Autodesk Fusion 360 part; units mm, degrees
note: some values were not read from the file. Set by a fixed rule: which sketch regions a step uses.
(part 3 of 4)
sketch "Sketch1" plane through (0, 0, 0) normal (0, 1, 0) x (1, 0, 0) in component "Laser"
  line L0 (18.5, 76) -> (18.5, 71)
  line L1 (18.5, 71) -> (33.5, 71)
  line L2 (33.5, 71) -> (33.5, 76)
  line L3 (33.5, 76) -> (18.5, 76)
  circle A0 centre (44, 73.5) radius 3.5355
  circle A1 centre (14, 13) radius 3.5355
  line L4 (3, 87.5) -> (3, 72.5)
  line L5 (3, 72.5) -> (8, 72.5)
  line L6 (8, 72.5) -> (8, 87.5)
  line L7 (8, 87.5) -> (3, 87.5)
  line L8 (3, 37.5) -> (3, 19.5)
  line L9 (3, 19.5) -> (8, 19.5)
  line L10 (8, 19.5) -> (8, 37.5)
  line L11 (8, 37.5) -> (3, 37.5)
  line L12 (46.0207, 66) -> (42.2092, 66)
  arc A2 (42.2092, 66) -> (38.5894, 63.702) centre (42.2092, 62) ccw
  line L13 (38.5894, 63.702) -> (18.9309, 21.8917)
  arc A3 (18.9309, 21.8917) -> (19.0866, 18.1897) centre (22.5507, 20.1897) ccw
  line L14 (19.0866, 18.1897) -> (20.9282, 15)
  arc A4 (20.9282, 11) -> (20.9282, 15) centre (17.4641, 13) ccw
  line L15 (20.9282, 11) -> (19.1962, 8)
  arc A5 (15.7321, 6) -> (19.1962, 8) centre (15.7321, 10) ccw
  line L16 (15.7321, 6) -> (3, 6)
  arc A6 (0, 9) -> (3, 6) centre (3, 9) ccw
  line L17 (0, 9) -> (0, 42)
  arc A7 (1, 43) -> (0, 42) centre (1, 42) ccw
  arc A8 (1, 43) -> (3, 45) centre (1, 45) ccw
  line L18 (3, 45) -> (3, 66)
  arc A9 (3, 66) -> (1, 68) centre (1, 66) ccw
  arc A10 (0, 69) -> (1, 68) centre (1, 69) ccw
  line L19 (0, 69) -> (0, 103)
  arc A11 (3, 106) -> (0, 103) centre (3, 103) ccw
  line L20 (8, 106) -> (3, 106)
  line L21 (8, 106) -> (11.4183, 106)
  arc A12 (14.1539, 104.9183) -> (11.4183, 106) centre (11.4183, 102) ccw
  line L22 (14.1539, 104.9183) -> (38.5159, 82.0817)
  arc A13 (38.5159, 82.0817) -> (41.2515, 81) centre (41.2515, 85) ccw
  line L23 (41.2515, 81) -> (46.0207, 81)
  arc A14 (49.4848, 79) -> (46.0207, 81) centre (46.0207, 77) ccw
  line L24 (49.4848, 79) -> (51.5056, 75.5)
  arc A15 (51.5056, 71.5) -> (51.5056, 75.5) centre (48.0415, 73.5) ccw
  line L25 (51.5056, 71.5) -> (49.4848, 68)
  arc A16 (46.0207, 66) -> (49.4848, 68) centre (46.0207, 70) ccw
  line L26 (40.0053, -0.251) -> (40.0053, -5.251)
  line L27 (40.0053, -5.251) -> (25.0053, -5.251)
  line L28 (25.0053, -5.251) -> (25.0053, -0.251)
  line L29 (25.0053, -0.251) -> (40.0053, -0.251)
  circle A17 centre (14.5053, -2.751) radius 3.5355
  circle A18 centre (44.5053, 57.749) radius 3.5355
  line L30 (55.5053, -1.751) -> (55.5053, -16.751)
  line L31 (55.5053, -16.751) -> (50.5053, -16.751)
  line L32 (50.5053, -16.751) -> (50.5053, -1.751)
  line L33 (50.5053, -1.751) -> (55.5053, -1.751)
  line L34 (55.5053, 51.249) -> (55.5053, 33.249)
  line L35 (55.5053, 33.249) -> (50.5053, 33.249)
  line L36 (50.5053, 33.249) -> (50.5053, 51.249)
  line L37 (50.5053, 51.249) -> (55.5053, 51.249)
  line L38 (16.296, 4.749) -> (12.4845, 4.749)
  arc A19 (12.4845, 4.749) -> (9.0204, 2.749) centre (12.4845, 0.749) ccw
  line L39 (9.0204, 2.749) -> (6.9997, -0.751)
  arc A20 (6.9997, -0.751) -> (6.9997, -4.751) centre (10.4638, -2.751) ccw
  line L40 (6.9997, -4.751) -> (9.0204, -8.251)
  arc A21 (9.0204, -8.251) -> (12.4845, -10.251) centre (12.4845, -6.251) ccw
  line L41 (12.4845, -10.251) -> (17.2537, -10.251)
  arc A22 (19.9893, -11.3327) -> (17.2537, -10.251) centre (17.2537, -14.251) ccw
  line L42 (19.9893, -11.3327) -> (44.3513, -34.1693)
  arc A23 (44.3513, -34.1693) -> (47.0869, -35.251) centre (47.0869, -31.251) ccw
  line L43 (47.0869, -35.251) -> (50.5053, -35.251)
  line L44 (50.5053, -35.251) -> (55.5053, -35.251)
  arc A24 (55.5053, -35.251) -> (58.5053, -32.251) centre (55.5053, -32.251) ccw
  line L45 (58.5053, -32.251) -> (58.5053, 1.749)
  arc A25 (58.5053, 1.749) -> (57.5053, 2.749) centre (57.5053, 1.749) ccw
  arc A26 (55.5053, 4.749) -> (57.5053, 2.749) centre (57.5053, 4.749) ccw
  line L46 (55.5053, 4.749) -> (55.5053, 25.749)
  arc A27 (57.5053, 27.749) -> (55.5053, 25.749) centre (57.5053, 25.749) ccw
  arc A28 (57.5053, 27.749) -> (58.5053, 28.749) centre (57.5053, 28.749) ccw
  line L47 (58.5053, 28.749) -> (58.5053, 61.749)
  arc A29 (58.5053, 61.749) -> (55.5053, 64.749) centre (55.5053, 61.749) ccw
  line L48 (55.5053, 64.749) -> (42.7732, 64.749)
  arc A30 (42.7732, 64.749) -> (39.3091, 62.749) centre (42.7732, 60.749) ccw
  line L49 (39.3091, 62.749) -> (37.5771, 59.749)
  arc A31 (37.5771, 59.749) -> (37.5771, 55.749) centre (41.0412, 57.749) ccw
  line L50 (37.5771, 55.749) -> (39.4186, 52.5593)
  arc A32 (39.5744, 48.8573) -> (39.4186, 52.5593) centre (35.9545, 50.5593) ccw
  line L51 (39.5744, 48.8573) -> (19.9159, 7.047)
  arc A33 (16.296, 4.749) -> (19.9159, 7.047) centre (16.296, 8.749) ccw
  line L52 (-16.3164, 46.5423) -> (-30.7017, 46.5423)
  arc A34 (-16.3164, 46.5423) -> (-13.3678, 50.0951) centre (-16.3164, 49.5423) ccw
  line L53 (-15.2428, 60.0951) -> (-13.3678, 50.0951)
  arc A35 (-15.2428, 60.0951) -> (-18.1914, 62.5423) centre (-18.1914, 59.5423) ccw
  line L54 (-30.7017, 62.5423) -> (-18.1914, 62.5423)
  line L55 (-43.2119, 62.5423) -> (-30.7017, 62.5423)
  arc A36 (-43.2119, 62.5423) -> (-46.1605, 60.0951) centre (-43.2119, 59.5423) ccw
  line L56 (-48.0355, 50.0951) -> (-46.1605, 60.0951)
  arc A37 (-48.0355, 50.0951) -> (-45.0869, 46.5423) centre (-45.0869, 49.5423) ccw
  line L57 (-30.7017, 46.5423) -> (-45.0869, 46.5423)
  line L58 (-42.2017, 41.5423) -> (-42.2017, 36.5423)
  line L59 (-42.2017, 36.5423) -> (-19.2017, 36.5423)
  line L60 (-19.2017, 36.5423) -> (-19.2017, 41.5423)
  line L61 (-19.2017, 41.5423) -> (-42.2017, 41.5423)
  line L62 (-55.7017, 94.5423) -> (-55.7017, 106.5423)
  line L63 (-55.7017, 106.5423) -> (-47.7017, 106.5423)
  line L64 (-45.7017, 104.5423) -> (-45.7017, 97.6156)
  line L65 (-44.8073, 95.949) -> (-31.8073, 87.3248)
  line L66 (-29.596, 87.3248) -> (-16.596, 95.949)
  line L67 (-15.7017, 97.6156) -> (-15.7017, 104.5423)
  line L68 (-13.7017, 106.5423) -> (-5.7178, 106.5423)
  line L69 (-5.7178, 106.5423) -> (-5.7017, 94.5423)
  line L70 (-5.7017, 94.5423) -> (-5.7017, 93.0423)
  line L71 (-5.7017, 93.0423) -> (-0.7017, 93.0423)
  line L72 (-0.7017, 93.0423) -> (-0.7017, 75.0423)
  line L73 (-0.7017, 75.0423) -> (-5.7017, 75.0423)
  line L74 (-5.7017, 75.0423) -> (-5.7017, 40.0423)
  line L75 (-5.7017, 40.0423) -> (-0.7017, 40.0423)
  line L76 (-0.7017, 40.0423) -> (-0.7017, 25.0423)
  line L77 (-0.7017, 25.0423) -> (-5.7017, 25.0423)
  line L78 (-5.7017, 25.0423) -> (-5.7017, 6.5423)
  line L79 (-5.7017, 6.5423) -> (-55.7017, 6.5423)
  line L80 (-55.7017, 6.5423) -> (-55.7017, 25.0423)
  line L81 (-55.7017, 25.0423) -> (-60.7017, 25.0423)
  line L82 (-60.7017, 25.0423) -> (-60.7017, 40.0423)
  line L83 (-60.7017, 40.0423) -> (-55.7017, 40.0423)
  line L84 (-55.7017, 40.0423) -> (-55.7017, 75.0423)
  line L85 (-55.7017, 75.0423) -> (-60.7017, 75.0423)
  line L86 (-60.7017, 75.0423) -> (-60.7017, 93.0423)
  line L87 (-60.7017, 93.0423) -> (-55.7017, 93.0423)
  line L88 (-55.7017, 93.0423) -> (-55.7017, 94.5423)
  line L89 (-2.7161, 5.444) -> (-0.1384, 4.2894)
  line L90 (-0.1384, 4.2894) -> (4.8616, 4.2894)
  spline S0 degree 2 poles (5.8616, 3.3935) (5.8616, 4.2894) (4.8616, 4.2894) knots -112.214913 -112.214913 -112.214913 -110.644117 -110.644117 -110.644117 weights 1 0.707107 1
  line L91 (5.8616, 3.3935) -> (5.8616, 0.7057)
  spline S1 degree 2 poles (4.8616, -0.1902) (5.8616, -0.1902) (5.8616, 0.7057) knots -116.78571 -116.78571 -116.78571 -115.214913 -115.214913 -115.214913 weights 1 0.707107 1
  line L92 (4.8616, -0.1902) -> (-0.1384, -0.1902)
  line L93 (-0.1384, -0.1902) -> (-2.7161, -1.3448)
  spline S2 degree 2 poles (-3.6105, -1.534) (-3.1384, -1.534) (-2.7161, -1.3448) knots -125.594971 -125.594971 -125.594971 -124.667676 -124.667676 -124.667676 weights 1 0.973249 1
  line L94 (-3.6105, -1.534) -> (-11.1384, -1.534)
  spline S3 degree 2 poles (-13.1384, -3.3258) (-13.1384, -1.534) (-11.1384, -1.534) knots -136.264428 -136.264428 -136.264428 -133.122835 -133.122835 -133.122835 weights 1 0.707107 1
  line L95 (-13.1384, -3.3258) -> (-13.1384, -8.7012)
  spline S4 degree 2 poles (-15.1384, -10.493) (-13.1384, -10.493) (-13.1384, -8.7012) knots -145.40602 -145.40602 -145.40602 -142.264428 -142.264428 -142.264428 weights 1 0.707107 1
  line L96 (-15.1384, -10.493) -> (-35.1384, -10.493)
  spline S5 degree 2 poles (-37.1384, -8.7012) (-37.1384, -10.493) (-35.1384, -10.493) knots -9.783185 -9.783185 -9.783185 -6.641593 -6.641593 -6.641593 weights 1 0.707107 1
  line L97 (-37.1384, -8.7012) -> (-37.1384, -3.3258)
  spline S6 degree 2 poles (-39.1384, -1.534) (-37.1384, -1.534) (-37.1384, -3.3258) knots -18.924778 -18.924778 -18.924778 -15.783185 -15.783185 -15.783185 weights 1 0.707107 1
  line L98 (-39.1384, -1.534) -> (-46.6663, -1.534)
  spline S7 degree 2 poles (-47.5607, -1.3448) (-47.1384, -1.534) (-46.6663, -1.534) knots -27.379937 -27.379937 -27.379937 -26.452642 -26.452642 -26.452642 weights 1 0.973249 1
  line L99 (-47.5607, -1.3448) -> (-50.1384, -0.1902)
  line L100 (-50.1384, -0.1902) -> (-55.1384, -0.1902)
  spline S8 degree 2 poles (-56.1384, 0.7057) (-56.1384, -0.1902) (-55.1384, -0.1902) knots -36.8327 -36.8327 -36.8327 -35.261903 -35.261903 -35.261903 weights 1 0.707107 1
  line L101 (-56.1384, 0.7057) -> (-56.1384, 3.3935)
  spline S9 degree 2 poles (-55.1384, 4.2894) (-56.1384, 4.2894) (-56.1384, 3.3935) knots -41.403496 -41.403496 -41.403496 -39.8327 -39.8327 -39.8327 weights 1 0.707107 1
  line L102 (-55.1384, 4.2894) -> (-50.1384, 4.2894)
  line L103 (-50.1384, 4.2894) -> (-47.5607, 5.444)
  spline S10 degree 2 poles (-46.6663, 5.6332) (-47.1384, 5.6332) (-47.5607, 5.444) knots -50.212757 -50.212757 -50.212757 -49.285462 -49.285462 -49.285462 weights 1 0.973249 1
  line L104 (-46.6663, 5.6332) -> (-34.1384, 5.6332)
  spline S11 degree 2 poles (-32.1384, 3.8414) (-32.1384, 5.6332) (-34.1384, 5.6332) knots -65.882214 -65.882214 -65.882214 -62.740621 -62.740621 -62.740621 weights 1 0.707107 1
  line L105 (-32.1384, 3.8414) -> (-32.1384, 0.2578)
  line L106 (-32.1384, 0.2578) -> (-18.1384, 0.2578)
  line L107 (-18.1384, 0.2578) -> (-18.1384, 3.8414)
  spline S12 degree 2 poles (-16.1384, 5.6332) (-18.1384, 5.6332) (-18.1384, 3.8414) knots -89.306992 -89.306992 -89.306992 -86.165399 -86.165399 -86.165399 weights 1 0.707107 1
  line L108 (-16.1384, 5.6332) -> (-3.6105, 5.6332)
  spline S13 degree 2 poles (-2.7161, 5.444) (-3.1384, 5.6332) (-3.6105, 5.6332) knots -102.762151 -102.762151 -102.762151 -101.834856 -101.834856 -101.834856 weights 1 0.973249 1
  arc A38 (-40.8714, -17.6968) -> (-38.5209, -18.8326) centre (-38.5209, -15.8326) ccw
  line L109 (-38.5209, -18.8326) -> (-14.4202, -18.8326)
  arc A39 (-14.4202, -18.8326) -> (-12.0697, -17.6968) centre (-14.4202, -15.8326) ccw
  line L110 (-1.4705, -4.3326) -> (3.5295, -4.3326)
  line L111 (3.5295, -4.3326) -> (3.5295, -19.3326)
  line L112 (3.5295, -19.3326) -> (-1.4705, -19.3326)
  line L113 (-1.4705, -19.3326) -> (-1.4705, -29.8326)
  line L114 (-1.4705, -29.8326) -> (-14.9705, -29.8326)
  line L115 (-14.9705, -29.8326) -> (-14.9705, -34.8326)
  line L116 (-14.9705, -34.8326) -> (-37.9705, -34.8326)
  line L117 (-37.9705, -34.8326) -> (-37.9705, -29.8326)
  line L118 (-37.9705, -29.8326) -> (-51.4705, -29.8326)
  line L119 (-51.4705, -29.8326) -> (-51.4705, -19.3326)
  line L120 (-51.4705, -19.3326) -> (-56.4705, -19.3326)
  line L121 (-56.4705, -19.3326) -> (-56.4705, -4.3326)
  line L122 (-56.4705, -4.3326) -> (-51.4705, -4.3326)
  line L123 (-51.4705, -4.3326) -> (-51.4705, -2.497)
  line L124 (-51.4705, -2.497) -> (-49.8826, -2.497)
  line L125 (-49.8826, -2.497) -> (-40.8714, -17.6968)
  line L126 (-12.0697, -17.6968) -> (-2.8826, -2.497)
  line L127 (-2.8826, -2.497) -> (-1.4705, -2.497)
  line L128 (-1.4705, -2.497) -> (-1.4705, -4.3326)
  line L129 (24.5846, -33.7494) -> (32.307, -41.9317)
  arc A40 (24.5846, -33.7494) -> (21.1301, -35.1221) centre (23.1301, -35.1221) ccw
  line L130 (21.1301, -43.3044) -> (21.1301, -35.1221)
  arc A41 (21.1301, -43.3044) -> (23.1301, -45.3044) centre (23.1301, -43.3044) ccw
  line L131 (30.8524, -45.3044) -> (23.1301, -45.3044)
  arc A42 (30.8524, -45.3044) -> (32.307, -41.9317) centre (30.8524, -43.3044) ccw
  arc A43 (-11.9711, -41.4934) -> (-11.1225, -45.3044) centre (-11.1225, -43.3044) ccw
  line L132 (-2.6294, -45.3044) -> (-11.1225, -45.3044)
  arc A44 (-2.6294, -45.3044) -> (-1.9491, -41.4237) centre (-2.6294, -43.3044) ccw
  line L133 (-6.7423, -39.69) -> (-1.9491, -41.4237)
  arc A45 (-6.7423, -39.69) -> (-8.2711, -39.7597) centre (-7.4225, -41.5707) ccw
  line L134 (-11.9711, -41.4934) -> (-8.2711, -39.7597)
  line L135 (13.4498, -41.6765) -> (3.4244, -38.0502)
  arc A46 (13.4498, -41.6765) -> (16.1301, -39.7957) centre (14.1301, -39.7957) ccw
  line L136 (16.1301, -31.4719) -> (16.1301, -39.7957)
  arc A47 (16.1301, -31.4719) -> (13.2815, -29.6609) centre (14.1301, -31.4719) ccw
  line L137 (3.256, -34.3584) -> (13.2815, -29.6609)
  arc A48 (3.256, -34.3584) -> (3.4244, -38.0502) centre (4.1046, -36.1695) ccw
  line L138 (-8.2711, -55.8492) -> (-11.9711, -54.1155)
  arc A49 (-8.2711, -55.8492) -> (-6.7423, -55.9189) centre (-7.4225, -54.0381) ccw
  line L139 (-1.9491, -54.1852) -> (-6.7423, -55.9189)
  arc A50 (-1.9491, -54.1852) -> (-2.6294, -50.3044) centre (-2.6294, -52.3044) ccw
  line L140 (-11.1225, -50.3044) -> (-2.6294, -50.3044)
  arc A51 (-11.1225, -50.3044) -> (-11.9711, -54.1155) centre (-11.1225, -52.3044) ccw
  arc A52 (13.2815, -65.948) -> (16.1301, -64.137) centre (14.1301, -64.137) ccw
  line L141 (16.1301, -55.8131) -> (16.1301, -64.137)
  arc A53 (16.1301, -55.8131) -> (13.4498, -53.9324) centre (14.1301, -55.8131) ccw
  line L142 (3.4244, -57.5586) -> (13.4498, -53.9324)
  arc A54 (3.4244, -57.5586) -> (3.256, -61.2504) centre (4.1046, -59.4394) ccw
  line L143 (13.2815, -65.948) -> (3.256, -61.2504)
  line L144 (21.1301, -60.4867) -> (21.1301, -52.3044)
  arc A55 (21.1301, -60.4867) -> (24.5846, -61.8595) centre (23.1301, -60.4867) ccw
  line L145 (32.307, -53.6772) -> (24.5846, -61.8595)
  arc A56 (32.307, -53.6772) -> (30.8524, -50.3044) centre (30.8524, -52.3044) ccw
  line L146 (23.1301, -50.3044) -> (30.8524, -50.3044)
  arc A57 (23.1301, -50.3044) -> (21.1301, -52.3044) centre (23.1301, -52.3044) ccw
  circle A58 centre (-35.1347, -47.8044) radius 0.375
  spline S14 degree 2 poles (20.1301, -78.8044) (21.1301, -78.8044) (21.1301, -77.8044) (21.1301, -75.3044) (21.1301, -72.8044) knots -186.864147 -186.864147 -186.864147 -185.29335 -185.29335 -180.29335 -180.29335 -180.29335 weights 1 0.707107 1 1 1
  line L147 (20.1301, -78.8044) -> (17.177, -78.8044)
  line L148 (17.1301, -78.8044) -> (17.177, -78.8044)
  spline S15 degree 2 poles (17.1301, -16.8044) (16.1301, -16.8044) (16.1301, -17.8044) (16.1301, -20.3044) (16.1301, -22.8044) knots -57.72942 -57.72942 -57.72942 -56.158624 -56.158624 -51.158624 -51.158624 -51.158624 weights 1 0.707107 1 1 1
  line L149 (20.1301, -16.8044) -> (17.1301, -16.8044)
  spline S16 degree 2 poles (21.1301, -22.8044) (21.1301, -20.3044) (21.1301, -17.8044) (21.1301, -16.8044) (20.1301, -16.8044) knots -67.300216 -67.300216 -67.300216 -62.300216 -62.300216 -60.72942 -60.72942 -60.72942 weights 1 1 1 0.707107 1
  spline S17 degree 2 poles (21.1301, -72.8044) (30.0204, -63.3846) (38.9108, -53.9647) (39.8424, -52.9775) (41.1039, -53.4788) (42.3653, -53.9801) (42.3653, -55.3374) (42.3653, -56.5709) (42.3653, -57.8044) (42.3653, -58.8044) (43.3653, -58.8044) (44.8653, -58.8044) (46.3653, -58.8044) (47.3653, -58.8044) (47.3653, -57.8044) (47.3653, -55.0544) (47.3653, -52.3044) (47.3653, -50.3044) (49.3653, -50.3044) (52.1153, -50.3044) (54.8653, -50.3044) (55.8653, -50.3044) (55.8653, -49.3044) (55.8653, -47.8044) (55.8653, -46.3044) (55.8653, -45.3044) (54.8653, -45.3044) (52.1153, -45.3044) (49.3653, -45.3044) (47.3653, -45.3044) (47.3653, -43.3044) (47.3653, -40.5544) (47.3653, -37.8044) (47.3653, -36.8044) (46.3653, -36.8044) (44.8653, -36.8044) (43.3653, -36.8044) (42.3653, -36.8044) (42.3653, -37.8044) (42.3653, -39.0379) (42.3653, -40.2714) (42.3653, -41.6288) (41.1039, -42.1301) (39.8424, -42.6313) (38.9108, -41.6442) (30.0204, -32.2243) (21.1301, -22.8044) knots -180.29335 -180.29335 -180.29335 -154.387975 -154.387975 -152.002869 -152.002869 -149.617763 -149.617763 -147.150765 -147.150765 -145.579969 -145.579969 -142.579969 -142.579969 -141.009172 -141.009172 -135.509172 -135.509172 -132.36758 -132.36758 -126.86758 -126.86758 -125.296783 -125.296783 -122.296783 -122.296783 -120.725987 -120.725987 -115.225987 -115.225987 -112.084394 -112.084394 -106.584394 -106.584394 -105.013598 -105.013598 -102.013598 -102.013598 -100.442802 -100.442802 -97.975804 -97.975804 -95.590698 -95.590698 -93.205592 -93.205592 -67.300216 -67.300216 -67.300216 weights 1 1 1 0.827432 1 0.827432 1 1 1 0.707107 1 1 1 0.707107 1 1 1 0.707107 1 1 1 0.707107 1 1 1 0.707107 1 1 1 0.707107 1 1 1 0.707107 1 1 1 0.707107 1 1 1 0.827432 1 0.827432 1 1 1
  line L150 (-47.8995, -42.8044) -> (-45.3836, -42.8044)
  line L151 (-44.4198, -42.5569) -> (-35.8866, -37.8636)
  line L152 (-33.8798, -37.9095) -> (-26.7944, -42.2394)
  line L153 (-24.8917, -42.3386) -> (16.1301, -22.8044)
  spline S18 degree 2 poles (16.1301, -72.8044) (16.1301, -75.3044) (16.1301, -77.8044) (16.1301, -78.8044) (17.1301, -78.8044) knots -196.434943 -196.434943 -196.434943 -191.434943 -191.434943 -189.864147 -189.864147 -189.864147 weights 1 1 1 0.707107 1
  line L154 (-24.8917, -53.2703) -> (16.1301, -72.8044)
  line L155 (-33.8798, -57.6994) -> (-26.7944, -53.3694)
  line L156 (-44.4198, -53.052) -> (-35.8866, -57.7453)
  line L157 (-47.8995, -52.8044) -> (-45.3836, -52.8044)
  line L158 (-49.8995, -44.8044) -> (-49.8995, -50.8044)
  arc A59 (-44.4198, -53.052) -> (-45.3836, -52.8044) centre (-45.3836, -54.8044) ccw
  arc A60 (-45.3836, -42.8044) -> (-44.4198, -42.5569) centre (-45.3836, -40.8044) ccw
  arc A61 (-47.8995, -42.8044) -> (-49.8995, -44.8044) centre (-47.8995, -44.8044) ccw
  arc A62 (-33.8798, -37.9095) -> (-35.8866, -37.8636) centre (-34.9227, -39.616) ccw
  arc A63 (-26.7944, -42.2394) -> (-24.8917, -42.3386) centre (-25.7515, -40.5329) ccw
  arc A64 (-24.8917, -53.2703) -> (-26.7944, -53.3694) centre (-25.7515, -55.076) ccw
  arc A65 (-35.8866, -57.7453) -> (-33.8798, -57.6994) centre (-34.9227, -55.9928) ccw
  arc A66 (-49.8995, -50.8044) -> (-47.8995, -52.8044) centre (-47.8995, -50.8044) ccw
  line L159 (-48.7017, 18.4806) -> (-48.7017, 14.5423)
  line L160 (-46.7017, 12.5423) -> (-41.5819, 12.5423)
  line L161 (-40.3625, 16.1275) -> (-45.4822, 20.0658)
  line L162 (-47.7017, 83.6559) -> (-47.7017, 69.5423)
  line L163 (-45.7017, 67.5423) -> (-35.7017, 67.5423)
  line L164 (-33.7017, 69.5423) -> (-33.7017, 76.513)
  line L165 (-34.5392, 78.1405) -> (-44.5392, 85.2834)
  line L166 (-25.7017, 29.5423) -> (-25.7017, 21.6316)
  line L167 (-22.4738, 20.0529) -> (-12.3029, 27.9636)
  line L168 (-13.5307, 31.5423) -> (-23.7017, 31.5423)
  line L169 (-15.9211, 20.0658) -> (-21.0408, 16.1275)
  line L170 (-19.8214, 12.5423) -> (-14.7017, 12.5423)
  line L171 (-12.7017, 14.5423) -> (-12.7017, 18.4806)
  line L172 (-27.7017, 76.513) -> (-27.7017, 69.5423)
  line L173 (-25.7017, 67.5423) -> (-15.7017, 67.5423)
  line L174 (-13.7017, 69.5423) -> (-13.7017, 83.6559)
  line L175 (-16.8641, 85.2834) -> (-26.8641, 78.1405)
  line L176 (-49.1005, 27.9636) -> (-38.9295, 20.0529)
  line L177 (-35.7017, 21.6316) -> (-35.7017, 29.5423)
  line L178 (-37.7017, 31.5423) -> (-47.8726, 31.5423)
  arc A67 (-48.7017, 14.5423) -> (-46.7017, 12.5423) centre (-46.7017, 14.5423) ccw
  arc A68 (-41.5819, 12.5423) -> (-40.3625, 16.1275) centre (-41.5819, 14.5423) ccw
  arc A69 (-45.4822, 20.0658) -> (-48.7017, 18.4806) centre (-46.7017, 18.4806) ccw
  arc A70 (-47.7017, 69.5423) -> (-45.7017, 67.5423) centre (-45.7017, 69.5423) ccw
  arc A71 (-35.7017, 67.5423) -> (-33.7017, 69.5423) centre (-35.7017, 69.5423) ccw
  arc A72 (-33.7017, 76.513) -> (-34.5392, 78.1405) centre (-35.7017, 76.513) ccw
  arc A73 (-44.5392, 85.2834) -> (-47.7017, 83.6559) centre (-45.7017, 83.6559) ccw
  arc A74 (-25.7017, 21.6316) -> (-22.4738, 20.0529) centre (-23.7017, 21.6316) ccw
  arc A75 (-12.3029, 27.9636) -> (-13.5307, 31.5423) centre (-13.5307, 29.5423) ccw
  arc A76 (-23.7017, 31.5423) -> (-25.7017, 29.5423) centre (-23.7017, 29.5423) ccw
  arc A77 (-21.0408, 16.1275) -> (-19.8214, 12.5423) centre (-19.8214, 14.5423) ccw
  arc A78 (-14.7017, 12.5423) -> (-12.7017, 14.5423) centre (-14.7017, 14.5423) ccw
  arc A79 (-12.7017, 18.4806) -> (-15.9211, 20.0658) centre (-14.7017, 18.4806) ccw
  arc A80 (-27.7017, 69.5423) -> (-25.7017, 67.5423) centre (-25.7017, 69.5423) ccw
  arc A81 (-15.7017, 67.5423) -> (-13.7017, 69.5423) centre (-15.7017, 69.5423) ccw
  arc A82 (-13.7017, 83.6559) -> (-16.8641, 85.2834) centre (-15.7017, 83.6559) ccw
  arc A83 (-26.8641, 78.1405) -> (-27.7017, 76.513) centre (-25.7017, 76.513) ccw
  arc A84 (-38.9295, 20.0529) -> (-35.7017, 21.6316) centre (-37.7017, 21.6316) ccw
  arc A85 (-35.7017, 29.5423) -> (-37.7017, 31.5423) centre (-37.7017, 29.5423) ccw
  arc A86 (-47.8726, 31.5423) -> (-49.1005, 27.9636) centre (-47.8726, 29.5423) ccw
  arc A87 (-45.7017, 104.5423) -> (-47.7017, 106.5423) centre (-47.7017, 104.5423) ccw
  arc A88 (-45.7017, 97.6156) -> (-44.8073, 95.949) centre (-43.7017, 97.6156) ccw
  arc A89 (-31.8073, 87.3248) -> (-29.596, 87.3248) centre (-30.7017, 88.9914) ccw
  arc A90 (-16.596, 95.949) -> (-15.7017, 97.6156) centre (-17.7017, 97.6156) ccw
  arc A91 (-13.7017, 106.5423) -> (-15.7017, 104.5423) centre (-13.7017, 104.5423) ccw
  arc A92 (16.6636, 53.9448) -> (12, 52.6922) centre (14.5, 52.6922) ccw
  line L179 (12, 52.6922) -> (12, 31.0216)
  arc A93 (12, 31.0216) -> (16.7553, 29.943) centre (14.5, 31.0216) ccw
  line L180 (16.7553, 29.943) -> (22.431, 41.8102)
  arc A94 (22.431, 41.8102) -> (22.3392, 44.1414) centre (20.1756, 42.8888) ccw
  line L181 (22.3392, 44.1414) -> (16.6636, 53.9448)
  arc A95 (23.5394, 52.2182) -> (27.9834, 52.4625) centre (25.6988, 53.4779) ccw
  line L182 (27.9834, 52.4625) -> (32.4376, 62.4847)
  arc A96 (32.4376, 62.4847) -> (30.1531, 66) centre (30.1531, 63.5) ccw
  line L183 (30.1531, 66) -> (19.8526, 66)
  arc A97 (19.8526, 66) -> (17.6931, 62.2403) centre (19.8526, 63.5) ccw
  line L184 (17.6931, 62.2403) -> (23.5394, 52.2182)
  arc A98 (12, 83.5) -> (14.5, 81) centre (14.5, 83.5) ccw
  line L185 (14.5, 81) -> (26.1249, 81)
  arc A99 (26.1249, 81) -> (27.8243, 85.3336) centre (26.1249, 83.5) ccw
  line L186 (27.8243, 85.3336) -> (16.1994, 96.1079)
  arc A100 (16.1994, 96.1079) -> (12, 94.2743) centre (14.5, 94.2743) ccw
  line L187 (12, 94.2743) -> (12, 83.5)
  line L188 (41.8417, 16.8043) -> (36.1661, 26.6076)
  arc A101 (36.0743, 28.9389) -> (36.1661, 26.6076) centre (38.3296, 27.8602) ccw
  line L189 (36.0743, 28.9389) -> (41.7499, 40.8061)
  arc A102 (46.5053, 39.7274) -> (41.7499, 40.8061) centre (44.0053, 39.7274) ccw
  line L190 (46.5053, 39.7274) -> (46.5053, 18.0569)
  arc A103 (41.8417, 16.8043) -> (46.5053, 18.0569) centre (44.0053, 18.0569) ccw
  line L191 (34.9659, 18.5308) -> (40.8121, 8.5087)
  arc A104 (38.6527, 4.749) -> (40.8121, 8.5087) centre (38.6527, 7.249) ccw
  line L192 (38.6527, 4.749) -> (28.3522, 4.749)
  arc A105 (26.0676, 8.2644) -> (28.3522, 4.749) centre (28.3522, 7.249) ccw
  line L193 (26.0676, 8.2644) -> (30.5219, 18.2865)
  arc A106 (34.9659, 18.5308) -> (30.5219, 18.2865) centre (32.8064, 17.2711) ccw
  line L194 (46.5053, -12.751) -> (46.5053, -23.5253)
  arc A107 (42.3059, -25.3588) -> (46.5053, -23.5253) centre (44.0053, -23.5253) ccw
  line L195 (42.3059, -25.3588) -> (30.681, -14.5845)
  arc A108 (32.3804, -10.251) -> (30.681, -14.5845) centre (32.3804, -12.751) ccw
  line L196 (32.3804, -10.251) -> (44.0053, -10.251)
  arc A109 (46.5053, -12.751) -> (44.0053, -10.251) centre (44.0053, -12.751) ccw
  line L197 (-6.0029, 6.9715) -> (-55, 7) construction
  line L198 (-55, 7) -> (-54.9971, 12.0285) construction
  line L199 (-54.9971, 12.0285) -> (-6, 12) construction
  line L200 (-6, 12) -> (-6.0029, 6.9715) construction
  line L201 (-1.5502, -47.9713) -> (-1.5877, -47.8678)
  line L202 (-1.5877, -47.8678) -> (-1.4719, -47.8496)
  line L203 (-1.4719, -47.8496) -> (-1.5367, -47.7594)
  line L204 (-1.5367, -47.7594) -> (-1.4303, -47.7129)
  line L205 (-1.4303, -47.7129) -> (-1.5191, -47.642)
  line L206 (-1.5191, -47.642) -> (-1.4303, -47.5707)
  line L207 (-1.4303, -47.5707) -> (-1.5367, -47.5246)
  line L208 (-1.5367, -47.5246) -> (-1.4719, -47.4338)
  line L209 (-1.4719, -47.4338) -> (-1.5877, -47.4158)
  line L210 (-1.5877, -47.4158) -> (-1.5502, -47.3127)
  line L211 (-1.5502, -47.3127) -> (-1.6672, -47.324)
  line L212 (-1.6672, -47.324) -> (-1.6631, -47.2156)
  line L213 (-1.6631, -47.2156) -> (-1.7723, -47.2557)
  line L214 (-1.7723, -47.2557) -> (-1.8, -47.1504)
  line L215 (-1.8, -47.1504) -> (-1.8934, -47.216)
  line L216 (-1.8934, -47.216) -> (-1.9508, -47.1215)
  line L217 (-1.9508, -47.1215) -> (-2.0217, -47.208)
  line L218 (-2.0217, -47.208) -> (-2.1045, -47.1309)
  line L219 (-2.1045, -47.1309) -> (-2.1473, -47.232)
  line L220 (-2.1473, -47.232) -> (-2.2496, -47.1785)
  line L221 (-2.2496, -47.1785) -> (-2.2611, -47.2865)
  line L222 (-2.2611, -47.2865) -> (-2.3756, -47.2605)
  line L223 (-2.3756, -47.2605) -> (-2.3553, -47.3674)
  line L224 (-2.3553, -47.3674) -> (-2.473, -47.3709)
  line L225 (-2.473, -47.3709) -> (-2.4221, -47.4687)
  line L226 (-2.4221, -47.4687) -> (-2.5346, -47.501)
  line L227 (-2.5346, -47.501) -> (-2.457, -47.5826)
  line L228 (-2.457, -47.5826) -> (-2.5557, -47.642)
  line L229 (-2.5557, -47.642) -> (-2.457, -47.7012)
  line L230 (-2.457, -47.7012) -> (-2.5346, -47.7826)
  line L231 (-2.5346, -47.7826) -> (-2.4221, -47.8152)
  line L232 (-2.4221, -47.8152) -> (-2.473, -47.9131)
  line L233 (-2.473, -47.9131) -> (-2.3553, -47.9164)
  line L234 (-2.3553, -47.9164) -> (-2.3756, -48.0232)
  line L235 (-2.3756, -48.0232) -> (-2.2611, -47.9971)
  line L236 (-2.2611, -47.9971) -> (-2.2496, -48.1055)
  line L237 (-2.2496, -48.1055) -> (-2.1473, -48.0518)
  line L238 (-2.1473, -48.0518) -> (-2.1045, -48.1527)
  line L239 (-2.1045, -48.1527) -> (-2.0217, -48.0758)
  line L240 (-2.0217, -48.0758) -> (-1.9508, -48.1625)
  line L241 (-1.9508, -48.1625) -> (-1.8934, -48.0676)
  line L242 (-1.8934, -48.0676) -> (-1.8, -48.1336)
  line L243 (-1.8, -48.1336) -> (-1.7723, -48.0281)
  line L244 (-1.7723, -48.0281) -> (-1.6631, -48.0684)
  line L245 (-1.6631, -48.0684) -> (-1.6672, -47.9596)
  line L246 (-1.6672, -47.9596) -> (-1.5502, -47.9713)
  line L247 (-2.252, -46.9203) -> (-2.2019, -46.9133)
  line L248 (-2.2019, -46.9133) -> (-2.166, -46.907)
  line L249 (-2.166, -46.907) -> (-1.9846, -46.9019)
  line L250 (-1.9846, -46.9019) -> (-1.8055, -46.9328)
  line L251 (-1.8055, -46.9328) -> (-1.7707, -46.9441)
  line L252 (-1.7707, -46.9441) -> (-1.7485, -46.9508)
  line L253 (-1.7485, -46.9508) -> (-1.6305, -46.9992)
  line L254 (-1.6305, -46.9992) -> (-1.4746, -47.0762)
  line L255 (-1.4746, -47.0762) -> (-1.4332, -47.0971)
  line L256 (-1.4332, -47.0971) -> (-1.4111, -47.1084)
  line L257 (-1.4111, -47.1084) -> (-1.3451, -47.1436)
  line L258 (-1.3451, -47.1436) -> (-1.2879, -47.175)
  line L259 (-1.2879, -47.175) -> (-1.2416, -47.1982)
  line L260 (-1.2416, -47.1982) -> (-1.2008, -47.2148)
  line L261 (-1.2008, -47.2148) -> (-1.1869, -47.2197)
  line L262 (-1.1869, -47.2197) -> (-1.1623, -47.2287)
  line L263 (-1.1623, -47.2287) -> (-0.9057, -47.2801)
  line L264 (-0.9057, -47.2801) -> (-0.8793, -47.2812)
  line L265 (-0.8793, -47.2812) -> (-0.7868, -47.2812)
  line L266 (-0.7868, -47.2812) -> (-0.5756, -47.2853)
  line L267 (-0.5756, -47.2853) -> (-0.5756, -48.0803)
  line L268 (-0.5756, -48.0803) -> (-0.8482, -48.0781)
  line L269 (-0.8482, -48.0781) -> (-0.8822, -48.0795)
  line L270 (-0.8822, -48.0795) -> (-1.2161, -48.1305)
  line L271 (-1.2161, -48.1305) -> (-1.2486, -48.1393)
  line L272 (-1.2486, -48.1393) -> (-1.2494, -48.1396)
  line L273 (-1.2494, -48.1396) -> (-1.258, -48.143)
  line L274 (-1.258, -48.143) -> (-1.2611, -48.143)
  line L275 (-1.2611, -48.143) -> (-1.2818, -48.149)
  line L276 (-1.2818, -48.149) -> (-1.474, -48.243)
  line L277 (-1.474, -48.243) -> (-1.4914, -48.2555)
  line L278 (-1.4914, -48.2555) -> (-1.5191, -48.274)
  line L279 (-1.5191, -48.274) -> (-1.6662, -48.3498)
  line L280 (-1.6662, -48.3498) -> (-1.823, -48.4021)
  line L281 (-1.823, -48.4021) -> (-1.8555, -48.4088)
  line L282 (-1.8555, -48.4088) -> (-1.8803, -48.4135)
  line L283 (-1.8803, -48.4135) -> (-2.1307, -48.4135)
  line L284 (-2.1307, -48.4135) -> (-2.1555, -48.4088)
  line L285 (-2.1555, -48.4088) -> (-2.1758, -48.4049)
  line L286 (-2.1758, -48.4049) -> (-2.3686, -48.3334)
  line L287 (-2.3686, -48.3334) -> (-2.3865, -48.3232)
  line L288 (-2.3865, -48.3232) -> (-2.4074, -48.3115)
  line L289 (-2.4074, -48.3115) -> (-2.5873, -48.158)
  line L290 (-2.5873, -48.158) -> (-2.6021, -48.1393)
  line L291 (-2.6021, -48.1393) -> (-2.6332, -48.1041)
  line L292 (-2.6332, -48.1041) -> (-2.7084, -47.9824)
  line L293 (-2.7084, -47.9824) -> (-2.7707, -47.8066)
  line L294 (-2.7707, -47.8066) -> (-2.7873, -47.6211)
  line L295 (-2.7873, -47.6211) -> (-2.7695, -47.4793)
  line L296 (-2.7695, -47.4793) -> (-2.7558, -47.4342)
  line L297 (-2.7558, -47.4342) -> (-2.7459, -47.385)
  line L298 (-2.7459, -47.385) -> (-2.685, -47.243)
  line L299 (-2.685, -47.243) -> (-2.5619, -47.0857)
  line L300 (-2.5619, -47.0857) -> (-2.3975, -46.9727)
  line L301 (-2.3975, -46.9727) -> (-2.252, -46.9203)
  line L302 (-0.2473, -49.8932) -> (-0.2955, -49.8217)
  line L303 (-0.2955, -49.8217) -> (-0.3131, -49.7561)
  line L304 (-0.3131, -49.7561) -> (-0.3131, -45.6998)
  line L305 (-0.3131, -45.6998) -> (-0.2951, -45.6344)
  line L306 (-0.2951, -45.6344) -> (-0.2469, -45.5633)
  line L307 (-0.2469, -45.5633) -> (-0.1756, -45.5152)
  line L308 (-0.1756, -45.5152) -> (-0.11, -45.4977)
  line L309 (-0.11, -45.4977) -> (0.2143, -45.4977)
  line L310 (0.2143, -45.4977) -> (0.2347, -45.4978)
  line L311 (0.2347, -45.4978) -> (0.2963, -45.5139)
  line L312 (0.2963, -45.5139) -> (0.365, -45.5572)
  line L313 (0.365, -45.5572) -> (0.4138, -45.6221)
  line L314 (0.4138, -45.6221) -> (0.4349, -45.6822)
  line L315 (0.4349, -45.6822) -> (0.4369, -45.7025)
  line L316 (0.4369, -45.7025) -> (-0.0881, -45.7025)
  line L317 (-0.0881, -45.7025) -> (-0.0881, -45.74)
  line L318 (-0.0881, -45.74) -> (0.4369, -45.74)
  line L319 (0.4369, -45.74) -> (0.4369, -46.3025)
  line L320 (0.4369, -46.3025) -> (0.1744, -46.3025)
  line L321 (0.1744, -46.3025) -> (0.1744, -46.34)
  line L322 (0.1744, -46.34) -> (0.4369, -46.34)
  line L323 (0.4369, -46.34) -> (0.4369, -47.015)
  line L324 (0.4369, -47.015) -> (0.1744, -47.015)
  line L325 (0.1744, -47.015) -> (0.1744, -47.0525)
  line L326 (0.1744, -47.0525) -> (0.4369, -47.0525)
  line L327 (0.4369, -47.0525) -> (0.4369, -47.7088)
  line L328 (0.4369, -47.7088) -> (-0.0881, -47.7088)
  line L329 (-0.0881, -47.7088) -> (-0.0881, -47.7463)
  line L330 (-0.0881, -47.7463) -> (0.4369, -47.7463)
  line L331 (0.4369, -47.7463) -> (0.4369, -48.365)
  line L332 (0.4369, -48.365) -> (0.1744, -48.365)
  line L333 (0.1744, -48.365) -> (0.1744, -48.4025)
  line L334 (0.1744, -48.4025) -> (0.4369, -48.4025)
  line L335 (0.4369, -48.4025) -> (0.4369, -49.04)
  line L336 (0.4369, -49.04) -> (0.1744, -49.04)
  line L337 (0.1744, -49.04) -> (0.1744, -49.0775)
  line L338 (0.1744, -49.0775) -> (0.4369, -49.0775)
  line L339 (0.4369, -49.0775) -> (0.4369, -49.715)
  line L340 (0.4369, -49.715) -> (-0.0881, -49.715)
  line L341 (-0.0881, -49.715) -> (-0.0881, -49.7525)
  line L342 (-0.0881, -49.7525) -> (0.4369, -49.7525)
  line L343 (0.4369, -49.7525) -> (0.4352, -49.7734)
  line L344 (0.4352, -49.7734) -> (0.4141, -49.8344)
  line L345 (0.4141, -49.8344) -> (0.3649, -49.8998)
  line L346 (0.3649, -49.8998) -> (0.2951, -49.9434)
  line L347 (0.2951, -49.9434) -> (0.2326, -49.9592)
  line L348 (0.2326, -49.9592) -> (0.2119, -49.959)
  line L349 (0.2119, -49.959) -> (-0.1101, -49.959)
  line L350 (-0.1101, -49.959) -> (-0.1758, -49.9414)
  line L351 (-0.1758, -49.9414) -> (-0.2473, -49.8932)
  line L352 (2.415, -47.3424) -> (2.4762, -47.3439)
  line L353 (2.4762, -47.3439) -> (3.089, -47.3582)
  line L354 (3.089, -47.3582) -> (3.1504, -47.3596)
  line L355 (3.1504, -47.3596) -> (3.1504, -48.1121)
  line L356 (3.1504, -48.1121) -> (2.9461, -48.1105)
  line L357 (2.9461, -48.1105) -> (0.9037, -48.0932)
  line L358 (0.9037, -48.0932) -> (0.6994, -48.0912)
  line L359 (0.6994, -48.0912) -> (0.6994, -47.3098)
  line L360 (0.6994, -47.3098) -> (2.415, -47.3424)
  line L361 (7.9147, -48.8502) -> (7.8945, -48.8449)
  line L362 (7.8945, -48.8449) -> (7.8699, -48.8383)
  line L363 (7.8699, -48.8383) -> (7.6387, -48.7359)
  line L364 (7.6387, -48.7359) -> (7.6174, -48.7223)
  line L365 (7.6174, -48.7223) -> (7.5865, -48.7041)
  line L366 (7.5865, -48.7041) -> (7.4975, -48.643)
  line L367 (7.4975, -48.643) -> (7.4238, -48.5805)
  line L368 (7.4238, -48.5805) -> (7.3545, -48.5199)
  line L369 (7.3545, -48.5199) -> (7.2756, -48.4635)
  line L370 (7.2756, -48.4635) -> (7.2481, -48.4467)
  line L371 (7.2481, -48.4467) -> (7.2162, -48.4281)
  line L372 (7.2162, -48.4281) -> (6.8826, -48.2746)
  line L373 (6.8826, -48.2746) -> (6.8479, -48.2625)
  line L374 (6.8479, -48.2625) -> (6.8369, -48.2588)
  line L375 (6.8369, -48.2588) -> (6.8041, -48.2477)
  line L376 (6.8041, -48.2477) -> (6.7717, -48.2375)
  line L377 (6.7717, -48.2375) -> (6.7311, -48.2248)
  line L378 (6.7311, -48.2248) -> (6.6799, -48.2074)
  line L379 (6.6799, -48.2074) -> (6.6631, -48.2014)
  line L380 (6.6631, -48.2014) -> (6.6457, -48.1941)
  line L381 (6.6457, -48.1941) -> (6.4662, -48.143)
  line L382 (6.4662, -48.143) -> (6.4479, -48.14)
  line L383 (6.4479, -48.14) -> (6.4375, -48.1391)
  line L384 (6.4375, -48.1391) -> (6.3346, -48.1391)
  line L385 (6.3346, -48.1391) -> (6.3244, -48.14)
  line L386 (6.3244, -48.14) -> (5.2654, -48.1303)
  line L387 (5.2654, -48.1303) -> (5.2654, -47.4076)
  line L388 (5.2654, -47.4076) -> (5.3563, -47.4098)
  line L389 (5.3563, -47.4098) -> (6.2645, -47.4307)
  line L390 (6.2645, -47.4307) -> (6.3555, -47.4326)
  line L391 (6.3555, -47.4326) -> (6.3656, -47.434)
  line L392 (6.3656, -47.434) -> (6.4686, -47.434)
  line L393 (6.4686, -47.434) -> (6.4789, -47.4326)
  line L394 (6.4789, -47.4326) -> (6.492, -47.4312)
  line L395 (6.492, -47.4312) -> (6.5317, -47.4238)
  line L396 (6.5317, -47.4238) -> (6.5971, -47.4043)
  line L397 (6.5971, -47.4043) -> (6.6803, -47.3682)
  line L398 (6.6803, -47.3682) -> (6.7606, -47.3256)
  line L399 (6.7606, -47.3256) -> (6.7867, -47.3102)
  line L400 (6.7867, -47.3102) -> (6.8025, -47.301)
  line L401 (6.8025, -47.301) -> (6.9565, -47.199)
  line L402 (6.9565, -47.199) -> (6.9712, -47.1879)
  line L403 (6.9712, -47.1879) -> (7.0084, -47.158)
  line L404 (7.0084, -47.158) -> (7.1223, -47.0703)
  line L405 (7.1223, -47.0703) -> (7.3035, -46.9426)
  line L406 (7.3035, -46.9426) -> (7.5031, -46.8225)
  line L407 (7.5031, -46.8225) -> (7.657, -46.7473)
  line L408 (7.657, -46.7473) -> (7.7104, -46.7277)
  line L409 (7.7104, -46.7277) -> (7.7119, -46.7293)
  line L410 (7.7119, -46.7293) -> (7.7734, -46.7074)
  line L411 (7.7734, -46.7074) -> (8.093, -46.6555)
  line L412 (8.093, -46.6555) -> (8.4154, -46.6803)
  line L413 (8.4154, -46.6803) -> (8.4787, -46.6969)
  line L414 (8.4787, -46.6969) -> (8.5154, -46.707)
  line L415 (8.5154, -46.707) -> (8.624, -46.7451)
  line L416 (8.624, -46.7451) -> (8.7691, -46.8094)
  line L417 (8.7691, -46.8094) -> (8.8898, -46.883)
  line L418 (8.8898, -46.883) -> (8.95, -46.9371)
  line L419 (8.95, -46.9371) -> (8.9617, -46.9594)
  line L420 (8.9617, -46.9594) -> (8.9531, -46.9594)
  line L421 (8.9531, -46.9594) -> (8.9273, -46.9627)
  line L422 (8.9273, -46.9627) -> (8.9242, -46.9633)
  line L423 (8.9242, -46.9633) -> (8.0123, -47.1477)
  line L424 (8.0123, -47.1477) -> (7.9965, -47.1502)
  line L425 (7.9965, -47.1502) -> (7.951, -47.1709)
  line L426 (7.951, -47.1709) -> (7.9055, -47.2146)
  line L427 (7.9055, -47.2146) -> (7.8805, -47.2725)
  line L428 (7.8805, -47.2725) -> (7.8769, -47.3223)
  line L429 (7.8769, -47.3223) -> (7.8803, -47.3379)
  line L430 (7.8803, -47.3379) -> (8.0971, -48.2473)
  line L431 (8.0971, -48.2473) -> (8.1016, -48.2631)
  line L432 (8.1016, -48.2631) -> (8.1274, -48.3068)
  line L433 (8.1274, -48.3068) -> (8.1758, -48.3492)
  line L434 (8.1758, -48.3492) -> (8.2365, -48.3711)
  line L435 (8.2365, -48.3711) -> (8.2873, -48.3725)
  line L436 (8.2873, -48.3725) -> (8.3033, -48.3687)
  line L437 (8.3033, -48.3687) -> (9.2152, -48.1842)
  line L438 (9.2152, -48.1842) -> (9.216, -48.184)
  line L439 (9.216, -48.184) -> (9.2248, -48.1812)
  line L440 (9.2248, -48.1812) -> (9.2258, -48.1809)
  line L441 (9.2258, -48.1809) -> (9.2207, -48.1902)
  line L442 (9.2207, -48.1902) -> (9.1625, -48.284)
  line L443 (9.1625, -48.284) -> (9.1557, -48.2934)
  line L444 (9.1557, -48.2934) -> (9.1439, -48.3098)
  line L445 (9.1439, -48.3098) -> (9.0158, -48.4633)
  line L446 (9.0158, -48.4633) -> (9.0019, -48.4775)
  line L447 (9.0019, -48.4775) -> (8.9773, -48.5033)
  line L448 (8.9773, -48.5033) -> (8.8525, -48.6248)
  line L449 (8.8525, -48.6248) -> (8.7019, -48.7336)
  line L450 (8.7019, -48.7336) -> (8.6644, -48.7531)
  line L451 (8.6644, -48.7531) -> (8.6449, -48.7633)
  line L452 (8.6449, -48.7633) -> (8.4393, -48.8398)
  line L453 (8.4393, -48.8398) -> (8.418, -48.8449)
  line L454 (8.418, -48.8449) -> (8.3953, -48.8506)
  line L455 (8.3953, -48.8506) -> (8.1641, -48.8762)
  line L456 (8.1641, -48.8762) -> (8.1408, -48.8758)
  line L457 (8.1408, -48.8758) -> (8.0842, -48.8758)
  line L458 (8.0842, -48.8758) -> (7.9147, -48.8502)
  line L459 (8.176, -44.1666) -> (8.825, -44.7019)
  line L460 (8.825, -44.7019) -> (9.3603, -45.351)
  line L461 (9.3603, -45.351) -> (9.7646, -46.0957)
  line L462 (9.7646, -46.0957) -> (10.0201, -46.9189)
  line L463 (10.0201, -46.9189) -> (10.1094, -47.5816)
  line L464 (10.1094, -47.5816) -> (10.1094, -47.8025)
  line L465 (10.1094, -47.8025) -> (10.1092, -48.0234)
  line L466 (10.1092, -48.0234) -> (10.0199, -48.6861)
  line L467 (10.0199, -48.6861) -> (9.7645, -49.5092)
  line L468 (9.7645, -49.5092) -> (9.3601, -50.2537)
  line L469 (9.3601, -50.2537) -> (8.8246, -50.9025)
  line L470 (8.8246, -50.9025) -> (8.1758, -51.4379)
  line L471 (8.1758, -51.4379) -> (7.4309, -51.8422)
  line L472 (7.4309, -51.8422) -> (6.608, -52.0975)
  line L473 (6.608, -52.0975) -> (5.9453, -52.1865)
  line L474 (5.9453, -52.1865) -> (5.6381, -52.1865)
  line L475 (5.6381, -52.1865) -> (5.6381, -51.6848)
  line L476 (5.6381, -51.6848) -> (5.9199, -51.6848)
  line L477 (5.9199, -51.6848) -> (6.5065, -51.6061)
  line L478 (6.5065, -51.6061) -> (7.2352, -51.3799)
  line L479 (7.2352, -51.3799) -> (7.8943, -51.0221)
  line L480 (7.8943, -51.0221) -> (8.4687, -50.548)
  line L481 (8.4687, -50.548) -> (8.9428, -49.9736)
  line L482 (8.9428, -49.9736) -> (9.3006, -49.3144)
  line L483 (9.3006, -49.3144) -> (9.5268, -48.5857)
  line L484 (9.5268, -48.5857) -> (9.6057, -47.9992)
  line L485 (9.6057, -47.9992) -> (9.6057, -47.608)
  line L486 (9.6057, -47.608) -> (9.5268, -47.0215)
  line L487 (9.5268, -47.0215) -> (9.3006, -46.2928)
  line L488 (9.3006, -46.2928) -> (8.9428, -45.6336)
  line L489 (8.9428, -45.6336) -> (8.4687, -45.0592)
  line L490 (8.4687, -45.0592) -> (7.8943, -44.5852)
  line L491 (7.8943, -44.5852) -> (7.2352, -44.2273)
  line L492 (7.2352, -44.2273) -> (6.5065, -44.0012)
  line L493 (6.5065, -44.0012) -> (5.9199, -43.9223)
  line L494 (5.9199, -43.9223) -> (5.6381, -43.9223)
  line L495 (5.6381, -43.9223) -> (5.6381, -43.4176)
  line L496 (5.6381, -43.4176) -> (5.9453, -43.4176)
  line L497 (5.9453, -43.4176) -> (6.608, -43.5068)
  line L498 (6.608, -43.5068) -> (7.431, -43.7623)
  line L499 (7.431, -43.7623) -> (8.176, -44.1666)
  line L500 (5.64, -41.2973) -> (5.6471, -41.2973)
  line L501 (5.6471, -41.2973) -> (5.7027, -41.2924)
  line L502 (5.7027, -41.2924) -> (5.8117, -41.2924)
  line L503 (5.8117, -41.2924) -> (5.8047, -41.3879)
  line L504 (5.8047, -41.3879) -> (5.8555, -41.6799)
  line L505 (5.8555, -41.6799) -> (6.0302, -42.015)
  line L506 (6.0302, -42.015) -> (6.3123, -42.2668)
  line L507 (6.3123, -42.2668) -> (6.583, -42.3877)
  line L508 (6.583, -42.3877) -> (6.6773, -42.4041)
  line L509 (6.6773, -42.4041) -> (6.7714, -42.4207)
  line L510 (6.7714, -42.4207) -> (7.067, -42.3994)
  line L511 (7.067, -42.3994) -> (7.418, -42.2588)
  line L512 (7.418, -42.2588) -> (7.6965, -42.0035)
  line L513 (7.6965, -42.0035) -> (7.8437, -41.7463)
  line L514 (7.8437, -41.7463) -> (7.8697, -41.6539)
  line L515 (7.8697, -41.6539) -> (7.8832, -41.6588)
  line L516 (7.8832, -41.6588) -> (8.0186, -41.7082)
  line L517 (8.0186, -41.7082) -> (8.0322, -41.7133)
  line L518 (8.0322, -41.7133) -> (7.9926, -41.8006)
  line L519 (7.9926, -41.8006) -> (7.9398, -42.0924)
  line L520 (7.9398, -42.0924) -> (7.9887, -42.4672)
  line L521 (7.9887, -42.4672) -> (8.167, -42.8006)
  line L522 (8.167, -42.8006) -> (8.3797, -43.0072)
  line L523 (8.3797, -43.0072) -> (8.4627, -43.0551)
  line L524 (8.4627, -43.0551) -> (8.5455, -43.1031)
  line L525 (8.5455, -43.1031) -> (8.8307, -43.1846)
  line L526 (8.8307, -43.1846) -> (9.2086, -43.173)
  line L527 (9.2086, -43.173) -> (9.558, -43.0287)
  line L528 (9.558, -43.0287) -> (9.7848, -42.8377)
  line L529 (9.7848, -42.8377) -> (9.8408, -42.7598)
  line L530 (9.8408, -42.7598) -> (9.852, -42.7691)
  line L531 (9.852, -42.7691) -> (9.9619, -42.8629)
  line L532 (9.9619, -42.8629) -> (9.9728, -42.8723)
  line L533 (9.9728, -42.8723) -> (9.9057, -42.941)
  line L534 (9.9057, -42.941) -> (9.7564, -43.1973)
  line L535 (9.7564, -43.1973) -> (9.6744, -43.5664)
  line L536 (9.6744, -43.5664) -> (9.7281, -43.9408)
  line L537 (9.7281, -43.9408) -> (9.8576, -44.2076)
  line L538 (9.8576, -44.2076) -> (9.9193, -44.2811)
  line L539 (9.9193, -44.2811) -> (9.9809, -44.3545)
  line L540 (9.9809, -44.3545) -> (10.2213, -44.5285)
  line L541 (10.2213, -44.5285) -> (10.5807, -44.6465)
  line L542 (10.5807, -44.6465) -> (10.9584, -44.6299)
  line L543 (10.9584, -44.6299) -> (11.2367, -44.5273)
  line L544 (11.2367, -44.5273) -> (11.316, -44.4732)
  line L545 (11.316, -44.4732) -> (11.3234, -44.4859)
  line L546 (11.3234, -44.4859) -> (11.3953, -44.6107)
  line L547 (11.3953, -44.6107) -> (11.4023, -44.6232)
  line L548 (11.4023, -44.6232) -> (11.3158, -44.6648)
  line L549 (11.3158, -44.6648) -> (11.0879, -44.8545)
  line L550 (11.0879, -44.8545) -> (10.8844, -45.1734)
  line L551 (10.8844, -45.1734) -> (10.8068, -45.5437)
  line L552 (10.8068, -45.5437) -> (10.8371, -45.8387)
  line L553 (10.8371, -45.8387) -> (10.8699, -45.9287)
  line L554 (10.8699, -45.9287) -> (10.9025, -46.0189)
  line L555 (10.9025, -46.0189) -> (11.0689, -46.2644)
  line L556 (11.0689, -46.2644) -> (11.3664, -46.4982)
  line L557 (11.3664, -46.4982) -> (11.7271, -46.6121)
  line L558 (11.7271, -46.6121) -> (12.0236, -46.6109)
  line L559 (12.0236, -46.6109) -> (12.1166, -46.5871)
  line L560 (12.1166, -46.5871) -> (12.1191, -46.6016)
  line L561 (12.1191, -46.6016) -> (12.1439, -46.7432)
  line L562 (12.1439, -46.7432) -> (12.1463, -46.7574)
  line L563 (12.1463, -46.7574) -> (12.051, -46.767)
  line L564 (12.051, -46.767) -> (11.7723, -46.8676)
  line L565 (11.7723, -46.8676) -> (11.4725, -47.0977)
  line L566 (11.4725, -47.0977) -> (11.2732, -47.4189)
  line L567 (11.2732, -47.4189) -> (11.2012, -47.7064)
  line L568 (11.2012, -47.7064) -> (11.2012, -47.898)
  line L569 (11.2012, -47.898) -> (11.2732, -48.1853)
  line L570 (11.2732, -48.1853) -> (11.4725, -48.5066)
  line L571 (11.4725, -48.5066) -> (11.7723, -48.7369)
  line L572 (11.7723, -48.7369) -> (12.051, -48.8373)
  line L573 (12.051, -48.8373) -> (12.1463, -48.8469)
  line L574 (12.1463, -48.8469) -> (12.1439, -48.8613)
  line L575 (12.1439, -48.8613) -> (12.1191, -49.0027)
  line L576 (12.1191, -49.0027) -> (12.1166, -49.0168)
  line L577 (12.1166, -49.0168) -> (12.0236, -48.993)
  line L578 (12.0236, -48.993) -> (11.7271, -48.9918)
  line L579 (11.7271, -48.9918) -> (11.3662, -49.1051)
  line L580 (11.3662, -49.1051) -> (11.0687, -49.3389)
  line L581 (11.0687, -49.3389) -> (10.9021, -49.5844)
  line L582 (10.9021, -49.5844) -> (10.8695, -49.6744)
  line L583 (10.8695, -49.6744) -> (10.8367, -49.7646)
  line L584 (10.8367, -49.7646) -> (10.806, -50.0596)
  line L585 (10.806, -50.0596) -> (10.8834, -50.4299)
  line L586 (10.8834, -50.4299) -> (11.0867, -50.749)
  line L587 (11.0867, -50.749) -> (11.3146, -50.9389)
  line L588 (11.3146, -50.9389) -> (11.4012, -50.9803)
  line L589 (11.4012, -50.9803) -> (11.3941, -50.9932)
  line L590 (11.3941, -50.9932) -> (11.3223, -51.118)
  line L591 (11.3223, -51.118) -> (11.3148, -51.1303)
  line L592 (11.3148, -51.1303) -> (11.2357, -51.0764)
  line L593 (11.2357, -51.0764) -> (10.9574, -50.9738)
  line L594 (10.9574, -50.9738) -> (10.5797, -50.957)
  line L595 (10.5797, -50.957) -> (10.2203, -51.0748)
  line L596 (10.2203, -51.0748) -> (9.9801, -51.2486)
  line L597 (9.9801, -51.2486) -> (9.9186, -51.3219)
  line L598 (9.9186, -51.3219) -> (9.8568, -51.3953)
  line L599 (9.8568, -51.3953) -> (9.7271, -51.6619)
  line L600 (9.7271, -51.6619) -> (9.6732, -52.0361)
  line L601 (9.6732, -52.0361) -> (9.7549, -52.4055)
  line L602 (9.7549, -52.4055) -> (9.9039, -52.6617)
  line L603 (9.9039, -52.6617) -> (9.9709, -52.7303)
  line L604 (9.9709, -52.7303) -> (9.96, -52.7396)
  line L605 (9.96, -52.7396) -> (9.8496, -52.832)
  line L606 (9.8496, -52.832) -> (9.8385, -52.841)
  line L607 (9.8385, -52.841) -> (9.7824, -52.7633)
  line L608 (9.7824, -52.7633) -> (9.5559, -52.5719)
  line L609 (9.5559, -52.5719) -> (9.2066, -52.4271)
  line L610 (9.2066, -52.4271) -> (8.8285, -52.4152)
  line L611 (8.8285, -52.4152) -> (8.5434, -52.4965)
  line L612 (8.5434, -52.4965) -> (8.4605, -52.5443)
  line L613 (8.4605, -52.5443) -> (8.3776, -52.5924)
  line L614 (8.3776, -52.5924) -> (8.1646, -52.799)
  line L615 (8.1646, -52.799) -> (7.9861, -53.1324)
  line L616 (7.9861, -53.1324) -> (7.9369, -53.5074)
  line L617 (7.9369, -53.5074) -> (7.9894, -53.7992)
  line L618 (7.9894, -53.7992) -> (8.0291, -53.8865)
  line L619 (8.0291, -53.8865) -> (8.0156, -53.892)
  line L620 (8.0156, -53.892) -> (7.8806, -53.941)
  line L621 (7.8806, -53.941) -> (7.8672, -53.9457)
  line L622 (7.8672, -53.9457) -> (7.8414, -53.8535)
  line L623 (7.8414, -53.8535) -> (7.6943, -53.5961)
  line L624 (7.6943, -53.5961) -> (7.4158, -53.3402)
  line L625 (7.4158, -53.3402) -> (7.0648, -53.1992)
  line L626 (7.0648, -53.1992) -> (6.7691, -53.1775)
  line L627 (6.7691, -53.1775) -> (6.6748, -53.1939)
  line L628 (6.6748, -53.1939) -> (6.5803, -53.2105)
  line L629 (6.5803, -53.2105) -> (6.3096, -53.3314)
  line L630 (6.3096, -53.3314) -> (6.0274, -53.5832)
  line L631 (6.0274, -53.5832) -> (5.8524, -53.9185)
  line L632 (5.8524, -53.9185) -> (5.8016, -54.2105)
  line L633 (5.8016, -54.2105) -> (5.8088, -54.306)
  line L634 (5.8088, -54.306) -> (5.6381, -54.306)
  line L635 (5.6381, -54.306) -> (5.6381, -52.8912)
  line L636 (5.6381, -52.8912) -> (5.8543, -52.8912)
  line L637 (5.8543, -52.8912) -> (6.2445, -52.865)
  line L638 (6.2445, -52.865) -> (6.7496, -52.7879)
  line L639 (6.7496, -52.7879) -> (7.2373, -52.6625)
  line L640 (7.2373, -52.6625) -> (7.7047, -52.4916)
  line L641 (7.7047, -52.4916) -> (8.1494, -52.2773)
  line L642 (8.1494, -52.2773) -> (8.5689, -52.0225)
  line L643 (8.5689, -52.0225) -> (8.9605, -51.7295)
  line L644 (8.9605, -51.7295) -> (9.3219, -51.4012)
  line L645 (9.3219, -51.4012) -> (9.6502, -51.0398)
  line L646 (9.6502, -51.0398) -> (9.9432, -50.6482)
  line L647 (9.9432, -50.6482) -> (10.1978, -50.2287)
  line L648 (10.1978, -50.2287) -> (10.4121, -49.784)
  line L649 (10.4121, -49.784) -> (10.5832, -49.3166)
  line L650 (10.5832, -49.3166) -> (10.7086, -48.8289)
  line L651 (10.7086, -48.8289) -> (10.7857, -48.3238)
  line L652 (10.7857, -48.3238) -> (10.8121, -47.9336)
  line L653 (10.8121, -47.9336) -> (10.8121, -47.6736)
  line L654 (10.8121, -47.6736) -> (10.7857, -47.2834)
  line L655 (10.7857, -47.2834) -> (10.7086, -46.7783)
  line L656 (10.7086, -46.7783) -> (10.5832, -46.2908)
  line L657 (10.5832, -46.2908) -> (10.4121, -45.8232)
  line L658 (10.4121, -45.8232) -> (10.1978, -45.3785)
  line L659 (10.1978, -45.3785) -> (9.9432, -44.9592)
  line L660 (9.9432, -44.9592) -> (9.6502, -44.5676)
  line L661 (9.6502, -44.5676) -> (9.3219, -44.2062)
  line L662 (9.3219, -44.2062) -> (8.9605, -43.8779)
  line L663 (8.9605, -43.8779) -> (8.5689, -43.585)
  line L664 (8.5689, -43.585) -> (8.1494, -43.3301)
  line L665 (8.1494, -43.3301) -> (7.7047, -43.1158)
  line L666 (7.7047, -43.1158) -> (7.2373, -42.9449)
  line L667 (7.2373, -42.9449) -> (6.7496, -42.8195)
  line L668 (6.7496, -42.8195) -> (6.2445, -42.7424)
  line L669 (6.2445, -42.7424) -> (5.8543, -42.716)
  line L670 (5.8543, -42.716) -> (5.6381, -42.716)
  line L671 (5.6381, -42.716) -> (5.6381, -41.4766)
  line L672 (5.6381, -41.4766) -> (5.6395, -41.4617)
  line L673 (5.6395, -41.4617) -> (5.641, -41.3123)
  line L674 (5.641, -41.3123) -> (5.64, -41.2973)
  line L675 (3.9836, -40.8754) -> (3.9574, -40.8867)
  line L676 (3.9574, -40.8867) -> (3.9772, -40.8812)
  line L677 (3.9772, -40.8812) -> (4.1787, -40.85)
  line L678 (4.1787, -40.85) -> (4.1992, -40.8492)
  line L679 (4.1992, -40.8492) -> (4.9117, -40.8492)
  line L680 (4.9117, -40.8492) -> (4.9117, -41.2168)
  line L681 (4.9117, -41.2168) -> (3.4369, -41.2168)
  line L682 (3.4369, -41.2168) -> (3.4369, -40.79)